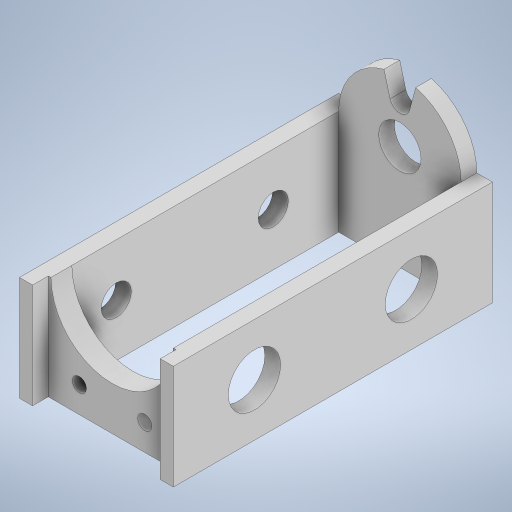
# Autodesk Inventor part: Xgantry_CableChain_top_connector
Saved by Autodesk Inventor 2023 (Build 270158000, 158)
## iProperties
Created: 2023-01-08
Part Number: Xgantry_CableChain_top_connector
Material: Generic
Document SubType Name: Modeling
Designer: a laptop
Density: 1 g/cm^3
Appearance: Default
Author: a laptop
Autodesk Inventor part; units mm, degrees
ref_plane "YZ Plane" through (0, 0, 0) normal (1, 0, 0) x (0, 1, 0)
ref_plane "XZ Plane" through (0, 0, 0) normal (0, 1, 0) x (-1, 0, 0)
ref_plane "XY Plane" through (0, 0, 0) normal (0, 0, 1) x (1, 0, 0)
sketch "Sketch1" plane through (0, 0, 0) normal (0, 0, 1) x (1, 0, 0)
  arc A0 (-1.9, 11.5447) -> (-3.0282, 11.3013) centre (0, 0) ccw construction
  line L0 (0, 7.75) -> (0, 0) construction
  arc A1 (1.9, 11.5447) -> (-1.9, 11.5447) centre (0, 0) ccw construction
  circle A2 centre (0, 0) radius 4.05
  line L1 (11.7, 0) -> (11.7, -20)
  line L2 (11.7, -20) -> (-11.7, -20)
  line L3 (-11.7, -20) -> (-11.7, 0)
  arc A3 (11.7, 0) -> (3.0282, 11.3013) centre (0, 0) ccw
  arc A4 (-11.7, 0) -> (11.7, 0) centre (0, 0) ccw construction
  line L4 (3.0282, 11.3013) -> (1.872, 6.9864)
  line L5 (-1.872, 6.9864) -> (-3.0282, 11.3013)
  arc A5 (-1.872, 6.9864) -> (1.872, 6.9864) centre (0, 7.488) ccw
  arc A6 (3.0282, 11.3013) -> (1.9, 11.5447) centre (0, 0) ccw construction
  arc A7 (-3.0282, 11.3013) -> (-11.7, 0) centre (0, 0) ccw
  line L6 (-1.872, 6.9864) -> (0, 0) construction
  line L7 (0, 0) -> (1.872, 6.9864) construction
  line L8 (0, 5.55) -> (0, 4.05) construction
  dimension "d3" = 8.1
  dimension "d0" = 23.4
  dimension "d4" = 20
  dimension "d8" = 30
  dimension "d9" = 1.5
  constraints: 18 end point, 17 point on circle, 7 centre point, 6 tangent, 3 coincident, 3 vertical, 2 collinear, 1 horizontal alignment, 1 parallel, 1 perpendicular, 1 point on line, 1 vertical alignment, 2 other
  measures "d0" diameter of A0
  measures "d4" distance from line of L2 point (0, 0)
  measures "d8" angle of L4 L5
  measures "d9" distance of L8.start L8.end
extrude "Extrusion1" add sketch "Sketch1" along normal blind 3
sketch "Sketch2" plane through (-11.7, -20, 0) normal (-1, 0, 0) x (0, 0, 1)
  line L0 (0, 20) -> (58, 20)
  line L1 (58, 20) -> (58, 0)
  line L2 (58, 0) -> (0, 0)
  line L3 (0, 0) -> (0, 20)
  line L4 (0, 0) -> (3, 0) projected
  line L5 (3, 20) -> (3, 0) projected
  dimension "d10" = 55
  constraints: 8 end point, 2 parallel, 1 horizontal, 1 perpendicular, 1 point on line
  measures "d10" distance between parallel lines of L1 L5
extrude "Extrusion2" add sketch "Sketch2" along normal blind 3
sketch "Sketch3" plane through (-11.7, -20, 58) normal (0, 0, 1) x (1, 0, 0)
  circle A0 centre (11.7, 20) radius 4.05 construction
  arc A1 (0, 20) -> (23.4, 20) centre (11.7, 20) ccw
  line L0 (23.4, 0) -> (23.4, 20) projected
  line L1 (23.4, 20) -> (23.4, 0)
  line L2 (23.4, 0) -> (0, 0)
  line L3 (23.4, 0) -> (-3, 0) construction
  line L4 (0, 0) -> (0, 20)
  constraints: 6 end point, 3 coincident, 2 point on circle, 1 centre point, 1 point on line, 1 vertical
extrude "Extrusion3" add sketch "Sketch3" against normal blind 4
sketch "Sketch4" plane through (-14.7, -20, 58) normal (0, 0, 1) x (1, 0, 0)
  circle A0 centre (8.45, 5) radius 1.35
  circle A1 centre (20.95, 5) radius 1.35
  line L0 (8.45, 5) -> (20.95, 5) construction
  line L1 (14.7, 5) -> (14.7, 20) construction
  dimension "d15" = 12.5
  dimension "d16" = 2.7
  dimension "d17" = 15
  constraints: 4 end point, 2 centre point, 1 equal radius, 1 horizontal, 1 midpoint, 1 perpendicular
  measures "d15" distance of L0.start L0.end
  measures "d16" diameter of A0
  measures "d17" distance of L1.start L1.end
extrude "Extrusion4" cut sketch "Sketch4" against normal up to surface (4 mm away)
sketch "Sketch5" plane through (11.7, -20, 0) normal (1, 0, 0) x (0, 0, -1)
  line L0 (0, 31.3013) -> (0, 20) construction
  line L1 (0, 20) -> (-58, 20)
  line L2 (-58, 20) -> (-58, 0)
  line L3 (-58, 0) -> (0, 0)
  line L4 (0, 0) -> (0, 20)
  constraints: 8 end point, 2 parallel, 1 horizontal, 1 perpendicular
extrude "Extrusion5" add sketch "Sketch5" along normal blind 3
sketch "Sketch7" plane through (-14.7, -20, 58) normal (0, 0, 1) x (1, 0, 0)
  line L0 (0, 20) -> (2.5, 20)
  line L1 (2.5, 20) -> (2.5, 0)
  line L2 (2.5, 0) -> (0, 0)
  line L3 (0, 0) -> (0, 20)
  line L4 (29.4, 20) -> (26.9, 20)
  line L5 (26.9, 20) -> (26.9, 0)
  line L6 (26.9, 0) -> (29.4, 0)
  line L7 (29.4, 0) -> (29.4, 20)
  point P0 (14.7, 20)
  dimension "d27" = 2.5
  constraints: 16 end point, 4 parallel, 3 point on line, 2 horizontal, 2 perpendicular, 1 collinear
  measures "d27" distance of L0.start L0.end
extrude "Extrusion7" add sketch "Sketch7" along normal blind 3
sketch "Sketch6" plane through (14.7, -20, 0) normal (1, 0, 0) x (0, 0, -1)
  line L0 (-45.5, 10) -> (-15.5, 10) construction
  line L1 (-58, 0) -> (0, 0) construction
  circle A0 centre (-45.5, 10) radius 2.8813
  circle A1 centre (-15.5, 10) radius 2.8813
  line L2 (0, 20) -> (-61, 20) construction
  line L3 (-30.5, 20) -> (-30.5, 10) construction
  dimension "d22" = 30
  dimension "d23" = 5.7625
  dimension "d24" = 10
  constraints: 4 end point, 2 centre point, 2 coincident, 2 midpoint, 1 equal radius, 1 horizontal, 1 perpendicular
  measures "d22" distance of L0.start L0.end
  measures "d23" diameter of A0
  measures "d24" distance between parallel lines of L1 L0
extrude "Extrusion6" cut sketch "Sketch6" against normal through all
sketch "Sketch8" plane through (14.7, -20, 0) normal (1, 0, 0) x (0, 0, -1)
  circle A0 centre (-15.5, 10) radius 5
  circle A1 centre (-45.5, 10) radius 5
  circle A2 centre (-15.5, 10) radius 2.8813 construction
  circle A3 centre (-45.5, 10) radius 2.8813 construction
  point P0 (0, 20)
  dimension "d30" = 10
  constraints: 2 centre point, 2 concentric, 1 equal radius
  measures "d30" diameter of A0
extrude "Extrusion8" cut sketch "Sketch8" against normal blind 3
body "Solid1"
